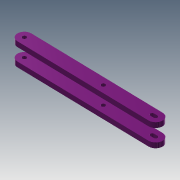
# Autodesk Inventor part: biela-dedo-3
Saved by Autodesk Inventor 2017 (Build 210142000, 142)
## iProperties
Created: 2018-05-30
Part Number: biela-dedo-3
Material: Generic
Document SubType Name: Modeling
Designer: Luiz Gustavo
Density: 1 g/cm^3
Appearance: Smooth - Purple
Mass: 9.61327 g
Surface Area: 72.187 cm^2
Volume: 9.61327 cm^3
Author: Luiz Gustavo
Autodesk Inventor part; units mm, degrees
ref_plane "YZ Plane" through (0, 0, 0) normal (1, 0, 0) x (0, 1, 0)
ref_plane "XZ Plane" through (0, 0, 0) normal (0, 1, 0) x (-1, 0, 0)
ref_plane "XY Plane" through (0, 0, 0) normal (0, 0, 1) x (1, 0, 0)
sketch "Sketch1" plane through (0, 0, 0) normal (0, 0, 1) x (1, 0, 0)
  line L0 (0, 0) -> (-64.457, 1.4619) construction
  line L1 (0, 0) -> (42.709, -0.9686) construction
  line L2 (40.3298, 14.0892) -> (39.9897, -0.907) construction
  circle A0 centre (-64.457, 1.4619) radius 1.55
  arc A1 (-64.5818, -4.0367) -> (-64.3323, 6.9605) centre (-64.457, 1.4619) ccw construction
  arc A2 (42.743, 0.531) -> (42.675, -2.4682) centre (42.709, -0.9686) ccw construction
  arc A3 (38.4901, -0.8729) -> (39.9557, -2.4066) centre (39.9897, -0.907) ccw
  arc A4 (42.8337, 4.53) -> (42.5843, -6.4672) centre (42.709, -0.9686) ccw construction
  line L3 (-64.3323, 6.9605) -> (42.8337, 4.53)
  line L4 (42.5843, -6.4672) -> (-64.5818, -4.0367)
  line L5 (42.743, 0.531) -> (40.0237, 0.5927)
  line L6 (42.675, -2.4682) -> (39.9557, -2.4066)
  arc A5 (42.675, -2.4682) -> (42.743, 0.531) centre (42.709, -0.9686) ccw
  arc A6 (40.0237, 0.5927) -> (38.4901, -0.8729) centre (39.9897, -0.907) ccw
  arc A7 (39.9557, -2.4066) -> (40.0237, 0.5927) centre (39.9897, -0.907) ccw construction
  arc A8 (42.5843, -6.4672) -> (42.8337, 4.53) centre (42.709, -0.9686) ccw
  arc A9 (-64.3323, 6.9605) -> (-64.5818, -4.0367) centre (-64.457, 1.4619) ccw
  circle A10 centre (0, 0) radius 1.55
  dimension "d0" = 3
  dimension "d1" = 11
  dimension "d13" = 3.1
  constraints: 18 point on circle, 11 centre point, 10 tangent, 8 end point, 6 coincident, 3 equal radius, 1 point on line
  measures "d0" diameter of A3
  measures "d1" diameter of A1
  measures "d13" diameter of A0
extrude "Extrusion1" add sketch "Sketch1" along normal mid plane 18
sketch "Sketch2" plane through (0, 0, 0) normal (0, 0, 1) x (1, 0, 0)
  arc A0 (42.675, -2.4682) -> (42.743, 0.531) centre (42.709, -0.9686) ccw projected
  line L0 (42.675, -2.4682) -> (39.9557, -2.4066) projected
  arc A1 (40.0237, 0.5927) -> (39.9557, -2.4066) centre (39.9897, -0.907) ccw projected
  line L1 (40.0237, 0.5927) -> (42.743, 0.531) projected
  circle A2 centre (0, 0) radius 1.55 projected
  circle A3 centre (-64.457, 1.4619) radius 1.55 projected
  line L2 (42.8337, 4.53) -> (-64.3323, 6.9605) projected
  arc A4 (-64.3323, 6.9605) -> (-64.5818, -4.0367) centre (-64.457, 1.4619) ccw projected
  line L3 (-64.5818, -4.0367) -> (42.5843, -6.4672) projected
  arc A5 (42.5843, -6.4672) -> (42.8337, 4.53) centre (42.709, -0.9686) ccw projected
extrude "Extrusion2" cut sketch "Sketch2" along normal mid plane 10
sketch "Sketch3" plane through (0, 0, 0) normal (0, 1, 0) x (-1, 0, 0)
  arc A0 (-43.8823, -9.7559) -> (-42.7176, -10.1422) centre (-40, 0) ccw
  line L0 (-40, 0) -> (0, 0) construction
  arc A1 (-43.8823, -14.4889) -> (-43.8823, 14.4889) centre (-40, 0) ccw construction
  line L1 (-40, 0) -> (-43.8823, -14.4889)
  line L2 (-40, 0) -> (-43.8823, 14.4889)
  line L3 (-43.8823, -14.4889) -> (-43.8823, 14.4889) construction
  arc A2 (-43.8823, 14.4889) -> (-43.8823, -14.4889) centre (-40, 0) ccw
  arc A3 (-43.8823, 9.7559) -> (-43.8823, -9.7559) centre (-40, 0) ccw
  arc A4 (-42.7176, -10.1422) -> (-42.7176, 10.1422) centre (-40, 0) ccw construction
  arc A5 (-42.7176, 10.1422) -> (-43.8823, 9.7559) centre (-40, 0) ccw
  dimension "d6" = 40
  dimension "d8" = 30
  dimension "d9" = 10.5
  dimension "d10" = 150
  constraints: 12 point on circle, 8 end point, 6 centre point, 4 point on line, 1 coincident, 1 horizontal, 1 vertical
  measures "d6" distance of L0.end L0.start
  measures "d8" diameter of A1
  measures "d9" radius of A4
  measures "d10" angle of L2 L1
extrude "Extrusion3" [suppressed]
body "Solid1"
